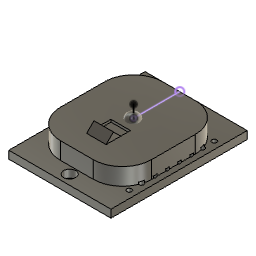
trackball-holder-mk6 v40 (Autodesk Fusion 360 archive; units mm, degrees)
design "PMW3360/3389"
Autodesk Fusion 360 part; units mm, degrees
sketch "Sketch1" plane through (0, 0, 0) normal (0, 0, 1) x (1, 0, 0)
  line L0 (0, 0) -> (0, 28) construction
  line L1 (0, 28) -> (21, 28) construction
  line L2 (21, 28) -> (0, 28) construction
  line L3 (0, 28) -> (0, 0) construction
  line L4 (0, 0) -> (21, 0) construction
  line L5 (21, 0) -> (21, 28) construction
  line L6 (10.5, 0) -> (10.5, 28) construction
  line L7 (10.5, 0) -> (10.5, 2) construction
  line L8 (10.5, 28) -> (10.5, 26) construction
  circle A0 centre (10.5, 26) radius 1.25 construction
  circle A1 centre (10.5, 2) radius 1.25 construction
  line L9 (21, 28) -> (0, 28)
  line L10 (0, 28) -> (0, 0)
  line L11 (0, 0) -> (21, 0)
  line L12 (21, 0) -> (21, 28)
  circle A2 centre (10.5, 2) radius 1.25
  circle A3 centre (10.5, 26) radius 1.25
  dimension "d38" = 28
  dimension "d39" = 21
  dimension "d40" = 2
  dimension "d41" = 2
  dimension "d42" = 2.5
  dimension "d43" = 2.5
  constraint coincident L0.start L3.end
  constraint vertical L0
  constraint perpendicular L0 L1
  constraint horizontal L2
  constraint vertical L3
  constraint horizontal L4
  constraint vertical L5
  constraint midpoint L4 L6.start
  constraint midpoint L2 L6.end
  constraint perpendicular L4 L7
  constraint perpendicular L1 L8
  constraint coincident L8.end A0.centre
  constraint coincident L7.end A1.centre
  constraint horizontal L9
  constraint vertical L10
  constraint horizontal L11
  constraint vertical L12
  constraint concentric A1 A2
  constraint concentric A0 A3
  measures "d38" distance of L0.start L0.end
  measures "d39" distance of L0.end L1.end
  measures "d40" distance of L6.start L7.end
  measures "d41" distance of L6.end L8.end
  measures "d42" diameter of A0
  measures "d43" diameter of A1
extrude "Extrude1" add sketch "Sketch1" along normal blind 1.6 makes body 1
sketch "Sketch2" plane through (0, 0, 1.6) normal (0, 0, 1) x (-1, 0, 0)
  circle A0 centre (-10.5, -26) radius 1.25
  circle A1 centre (-10.5, -2) radius 1.25
  line L0 (-21, 0) -> (-21, -28)
  line L1 (-21, -28) -> (0, -28)
  line L2 (0, -28) -> (0, 0)
  line L3 (0, 0) -> (-21, 0)
  line L4 (0, -14) -> (-21, -14) construction
  line L5 (-10.5, -28) -> (-10.5, 0) construction
  line L6 (-10.5, -14) -> (-10.5, -24.5) construction
  line L7 (-10.5, -24.5) -> (-19.85, -24.5) construction
  line L8 (-10.5, -14) -> (-10.5, -3.5) construction
  line L9 (-10.5, -3.5) -> (-1.15, -3.5) construction
  line L10 (-1.15, -3.5) -> (-19.85, -3.5) construction
  line L11 (-19.85, -3.5) -> (-19.85, -24.5) construction
  line L12 (-19.85, -24.5) -> (-1.15, -24.5) construction
  line L13 (-1.15, -24.5) -> (-1.15, -3.5) construction
  line L14 (-1.15, -3.5) -> (-19.85, -3.5)
  line L15 (-19.85, -3.5) -> (-19.85, -24.5)
  line L16 (-19.85, -24.5) -> (-1.15, -24.5)
  line L17 (-1.15, -24.5) -> (-1.15, -3.5)
  dimension "d46" = 10.5
  dimension "d47" = 9.35
  dimension "d48" = 10.5
  dimension "d49" = 9.35
  constraint midpoint L2 L4.start
  constraint midpoint L0 L4.end
  constraint midpoint L1 L5.start
  constraint midpoint L3 L5.end
  constraint midpoint L5 L6.start
  constraint perpendicular L4 L6
  constraint perpendicular L6 L7
  constraint perpendicular L7 L8
  constraint perpendicular L5 L9
  constraint horizontal L10
  constraint vertical L11
  constraint horizontal L12
  constraint vertical L13
  constraint horizontal L14
  constraint vertical L15
  constraint horizontal L16
  constraint vertical L17
  measures "d46" distance of L6.start L6.end
  measures "d47" distance of L6.end L7.end
  measures "d48" distance of L6.start L8.end
  measures "d49" distance of L8.end L9.end
extrude "Extrude2" add sketch "Sketch2" along normal blind 3.5 contours L14 L15 L16 L17 bodies 1
fillet "Fillet1" radius 6 4 edges at (19.85, 3.5, 3.35) (1.15, 3.5, 3.35) (1.15, 24.5, 3.35) (19.85, 24.5, 3.35) on bodies 1
sketch "Sketch3" plane through (0, 0, 5.1) normal (0, 0, 1) x (-1, 0, 0)
  arc A0 (-19.85, -18.5) -> (-13.85, -24.5) centre (-13.85, -18.5) ccw
  line L0 (-13.85, -24.5) -> (-7.15, -24.5)
  arc A1 (-7.15, -24.5) -> (-1.15, -18.5) centre (-7.15, -18.5) ccw
  line L1 (-1.15, -18.5) -> (-1.15, -9.5)
  arc A2 (-1.15, -9.5) -> (-7.15, -3.5) centre (-7.15, -9.5) ccw
  line L2 (-7.15, -3.5) -> (-13.85, -3.5)
  arc A3 (-13.85, -3.5) -> (-19.85, -9.5) centre (-13.85, -9.5) ccw
  line L3 (-19.85, -9.5) -> (-19.85, -18.5)
  line L4 (0, 0) -> (-21, 0)
  line L5 (-10.5, 0) -> (-10.5, -15)
  circle A4 centre (-10.5, -15) radius 1.5
  line L6 (-10.5, 0) -> (-10.5, -10.5)
  line L7 (-10.5, -10.5) -> (-12.5, -10.5)
  line L8 (-12.5, -10.5) -> (-12.5, -12.5)
  line L9 (-12.5, -12.5) -> (-8.5, -12.5)
  line L10 (-8.5, -12.5) -> (-8.5, -10.5)
  line L11 (-8.5, -10.5) -> (-12.5, -10.5)
  circle A5 centre (-10.5, -2) radius 1.25
  circle A6 centre (-10.5, -26) radius 1.25
  line L12 (-21, -28) -> (-21, 0)
  line L13 (-21, 0) -> (0, 0)
  line L14 (0, 0) -> (0, -28)
  line L15 (0, -28) -> (-21, -28)
  line L16 (-12.5, -10.5) -> (-12.5, -7.5)
  line L17 (-12.5, -7.5) -> (-8.5, -7.5)
  line L18 (-8.5, -7.5) -> (-8.5, -10.5)
  dimension "d1" = 15
  dimension "d2" = 3
  dimension "d3" = 10.5
  dimension "d4" = 2
  dimension "d5" = 2
  dimension "d6" = 4
  dimension "d7" = 2
  dimension "d11" = 3
  dimension "d12" = 4
  constraint midpoint L4 L5.start
  constraint perpendicular L4 L5
  constraint coincident L5.end A4.centre
  constraint perpendicular L4 L6
  constraint perpendicular L5 L7
  constraint perpendicular L7 L8
  constraint perpendicular L8 L9
  constraint perpendicular L9 L10
  constraint perpendicular L7 L16
  constraint perpendicular L16 L17
  measures "d1" distance of L5.start L5.end
  measures "d2" diameter of A4
  measures "d3" distance of L5.start L6.end
  measures "d4" distance of L6.end L7.end
  measures "d5" distance of L7.end L8.end
  measures "d6" distance of L8.end L9.end
  measures "d7" distance of L9.end L10.end
  measures "d11" distance of L7.end L16.end
  measures "d12" distance of L16.end L17.end
extrude "Extrude4" add sketch "Sketch3" along normal blind 1.5 contours L5 L6 L11 L17 L18 | L5 L6 L7 L11 L16 L17 bodies 1
extrude "Extrude3" cut sketch "Sketch3" against normal blind 0.5 contours L5 L9 L10 L11 | L5 L7 L8 L9 L11 bodies 1
sphere "SpherePrimitive1" add diameter 3 placed x (-1, 0, 0) y (0, -1, 0) z (0, 0, 1) at (10.5, 15, 5.1) separate body makes body 2
move_body "Move1" bodies 2 to x (1, 0, 0) y (0, 1, 0) z (0, 0, 1) at (0, 0, -0.5)
sketch "Sketch5" plane through (12.5, 0, 0) normal (1, 0, 0) x (0, 1, 0)
  line L0 (7.5, 5.1) -> (10.5, 5.1)
  line L1 (10.5, 5.1) -> (10.5, 6.6)
  line L2 (10.5, 6.6) -> (7.5, 6.6)
  line L3 (7.5, 6.6) -> (7.5, 5.1)
  line L4 (10.5, 5.1) -> (9, 6.6)
  line L5 (9, 6.6) -> (7.5, 5.1)
  constraint coincident L0.end L1.start
  constraint midpoint L2 L4.end
  constraint coincident L0.start L3.end
extrude "Extrude5" cut sketch "Sketch5" against normal blind 4 contours L2 L3 L5 | L1 L2 L4 bodies 1
sketch "Sketch6" plane through (0, 0, 0) normal (0, 0, -1) x (1, 0, 0)
  circle A0 centre (10.5, -2) radius 1.25
  circle A1 centre (10.5, -26) radius 1.25
  line L0 (21, -28) -> (21, 0)
  line L1 (21, 0) -> (0, 0)
  line L2 (0, 0) -> (0, -28)
  line L3 (0, -28) -> (21, -28)
  line L4 (1.5, -1.5) -> (1.5, -26.5)
  line L5 (1.5, -26.5) -> (19.5, -26.5)
  line L6 (19.5, -26.5) -> (19.5, -1.5)
  line L7 (19.5, -1.5) -> (1.5, -1.5)
  line L8 (19.5, -14) -> (19.5, -4)
  line L9 (19.5, -14) -> (19.5, -24)
  line L10 (19.5, -4) -> (19.5, -4.75)
  line L11 (19.5, -4.75) -> (19.5, -5.25)
  circle A2 centre (19.5, -5.25) radius 0.5
  line L12 (19.5, -5.75) -> (19.5, -7.75)
  circle A3 centre (19.5, -7.75) radius 0.5
  line L13 (19.5, -8.25) -> (19.5, -10.25)
  line L14 (19.5, -10.25) -> (19.5, -9.5)
  line L15 (19.5, -10.25) -> (19.5, -12.75)
  circle A4 centre (19.5, -10.25) radius 0.5
  circle A5 centre (19.5, -12.75) radius 0.5
  line L16 (19.5, -12.75) -> (19.5, -15.25)
  line L17 (19.5, -15.25) -> (19.5, -17.75)
  line L18 (19.5, -17.75) -> (19.5, -20.25)
  line L19 (19.5, -20.25) -> (19.5, -22.75)
  circle A6 centre (19.5, -15.25) radius 0.5
  circle A7 centre (19.5, -17.75) radius 0.5
  circle A8 centre (19.5, -20.25) radius 0.5
  circle A9 centre (19.5, -22.75) radius 0.5
  dimension "d17" = -1.5
  dimension "d18" = 10
  dimension "d19" = 10
  dimension "d20" = 0.75
  dimension "d21" = 0.5
  dimension "d22" = 1
  dimension "d23" = 2
  dimension "d24" = 1
  dimension "d25" = 2
  dimension "d26" = 2.5
  dimension "d27" = 1
  dimension "d28" = 1
  dimension "d29" = 2.5
  dimension "d30" = 2.5
  dimension "d31" = 2.5
  dimension "d32" = 2.5
  dimension "d33" = 1
  dimension "d34" = 1
  dimension "d35" = 1
  dimension "d36" = 1
  constraint midpoint L6 L8.start
  constraint parallel L6 L8
  constraint parallel L6 L9
  constraint parallel L6 L10
  constraint parallel L8 L11
  constraint coincident L11.end A2.centre
  constraint coincident L8 L12.start
  constraint coincident A2 L12.start
  constraint parallel L6 L12
  constraint coincident L12.end A3.centre
  constraint coincident A3 L13.start
  constraint coincident L6 L13.start
  constraint parallel L8 L13
  constraint coincident L6 L14.end
  constraint parallel L8 L15
  constraint coincident L13.end L14.start
  constraint coincident L15.end A5.centre
  constraint parallel L6 L16
  constraint parallel L9 L17
  constraint parallel L6 L18
  constraint parallel L6 L19
  constraint coincident L16.end L17.start
  constraint coincident L17.end L18.start
  constraint coincident L18.end L19.start
  constraint coincident L19.end A9.centre
  measures "d18" distance of L8.start L8.end
  measures "d19" distance of L8.start L9.end
  measures "d20" distance of L8.end L10.end
  measures "d21" distance of L10.end L11.end
  measures "d22" diameter of A2
  measures "d23" distance of L12.start L12.end
  measures "d24" diameter of A3
  measures "d25" distance of L13.start L13.end
  measures "d26" distance of L13.end L15.end
  measures "d27" diameter of A4
  measures "d28" diameter of A5
  measures "d29" distance of L15.end L16.end
  measures "d30" distance of L16.end L17.end
  measures "d31" distance of L17.end L18.end
  measures "d32" distance of L18.end L19.end
  measures "d33" diameter of A6
  measures "d34" diameter of A7
  measures "d35" diameter of A8
  measures "d36" diameter of A9
extrude "Extrude6" cut sketch "Sketch6" against normal blind 2 contours L6 L8 L11 A2 | L6 L8 L11 A2 | L6 L8 L12 A3 | L6 L8 L12 A3 | L6 L9 L19 A9 | L6 L9 L19 A9 | L6 L8 L13 L14 L15 A4 | L6 L8 L13 L14 L15 A4 | L6 L9 L18 L19 A8 | L6 L9 L18 L19 A8 | L6 L8 L15 A5 L16 | L6 L8 L15 A5 L16 | L6 L9 L17 L18 A7 | L6 L9 L17 L18 A7 | L6 L9 L16 L17 A6 | L6 L9 L16 L17 A6 bodies 1
sketch "Sketch1 (2)" plane through (0, 0, 5.1) normal (0, 0, 1) x (-1, 0, 0) in component "center-pointer"
  arc A0 (-19.85, -18.5) -> (-13.85, -24.5) centre (-13.85, -18.5) ccw
  line L0 (-13.85, -24.5) -> (-7.15, -24.5)
  arc A1 (-7.15, -24.5) -> (-1.15, -18.5) centre (-7.15, -18.5) ccw
  line L1 (-1.15, -18.5) -> (-1.15, -9.5)
  arc A2 (-1.15, -9.5) -> (-7.15, -3.5) centre (-7.15, -9.5) ccw
  line L2 (-7.15, -3.5) -> (-13.85, -3.5)
  arc A3 (-13.85, -3.5) -> (-19.85, -9.5) centre (-13.85, -9.5) ccw
  line L3 (-19.85, -9.5) -> (-19.85, -18.5)
  line L4 (-8.5, -10.5) -> (-8.5, -12.5)
  line L5 (-8.5, -12.5) -> (-12.5, -12.5)
  line L6 (-12.5, -12.5) -> (-12.5, -10.5)
  line L7 (-12.5, -10.5) -> (-12.5, -7.5)
  line L8 (-12.5, -7.5) -> (-8.5, -7.5)
  line L9 (-8.5, -7.5) -> (-8.5, -10.5)
  line L10 (-10.5, -24.5) -> (-10.5, -15)
  dimension "d55" = 9.5
  constraint midpoint L0 L10.start
  constraint perpendicular L0 L10
  measures "d55" distance of L10.start L10.end
ref_plane "WorkPlane1" through (10.65, 14, 3.35) normal (-1, 0, 0) x (0, -1, 0) in component "center-pointer"
sketch "Sketch2 (2)" plane through (10.65, 14, 3.35) normal (-1, 0, 0) x (0, 1, 0) in component "center-pointer"
  line L0 (10.5, -1.75) -> (1, -1.75)
  line L1 (1, -1.75) -> (1, -4.25)
  dimension "d57" = 2.5
  constraint coincident L0.end L1.start
  constraint perpendicular L0 L1
  measures "d57" distance of L0.end L1.end
component "center-pointer" placed x (1, 0, 0) y (0, 1, 0) z (0, 0, 1) at (0, 0, 0)

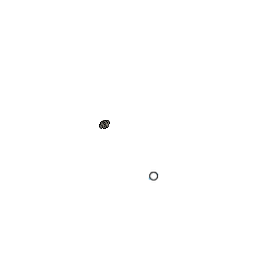
design "Mini-Bearing"
Autodesk Fusion 360 part; units mm, degrees
sketch "Sketch1" plane through (0, 0, 0) normal (0, 0, 1) x (1, 0, 0)
  circle A0 centre (0, 0) radius 3.5
  circle A1 centre (0, 0) radius 1.95
  dimension "d85" = 7
  dimension "d86" = 3.9
  constraint coincident A0.centre A1.centre
  measures "d85" diameter of A0
  measures "d86" diameter of A1
extrude "Extrude1" add sketch "Sketch1" along normal blind 2.5
sketch "Sketch2" plane through (0, 0, 0) normal (0, 0, 1) x (1, 0, 0)
  circle A0 centre (0, 0) radius 2
  constraint coincident A0.centre origin
extrude "Extrude2" add sketch "Sketch2" against normal blind 3
extrude "Extrude3" add 1 faces at (-0.325, 0.3213, 0) along direction (0, 0, 1) blind 5.5
move_body "Move1" bodies 1 to x (1, 0, 0) y (0, 1, 0) z (0, 0, 1) at (-1.4953, -0.1188, 0)
sketch "sketch 496" plane through (73.8903, -150.6507, -43.9901) normal (-0.866025, 0, 0.5) x (-0.5, 0, -0.866025)
  line L0 (-95.4904, -88.9756) -> (-91.7882, -86.9923)
  line L1 (-95.4904, -88.9756) -> (-91.7882, -86.9923)
  line L2 (-91.7882, -86.9923) -> (-92.5153, -85.635)
  arc A0 (-92.5153, -85.635) -> (-96.5133, -87.0663) centre (-93.3717, -89.5423) ccw
  line L3 (-95.4904, -88.9756) -> (-96.5133, -87.0663)
  line L4 (-89.6444, -90.994) -> (-90.3715, -89.6367)
  line L5 (-90.3715, -89.6367) -> (-94.0738, -91.6201)
  line L6 (-90.3715, -89.6367) -> (-94.0738, -91.6201)
  line L7 (-93.0509, -93.5294) -> (-94.0738, -91.6201)
  arc A1 (-93.0509, -93.5294) -> (-89.6444, -90.994) centre (-93.3717, -89.5423) ccw
  arc A2 (-93.0509, -93.5294) -> (-89.6444, -90.994) centre (-93.3717, -89.5423) ccw
extrude "Extrude4" cut sketch "sketch 496" against normal blind 5
move_body "Move2" bodies 1 to x (1, 0, 0) y (0, 0, 1) z (0, -1, 0) at (0, 2.3812, 2.6188)
move_body "Move3" bodies 1 to x (1, 0, 0) y (0, 1, 0) z (0, 0, 1) at (1.5, -1.1, -2.5)
ref_plane "WorkPlane1" through (1.9547, -2.6103, 0) normal (1, 0, 0) x (0, 0, -1)
ref_plane "WorkPlane2" through (0.0047, -2.6103, 0) normal (1, 0, 0) x (0, 0, -1)
